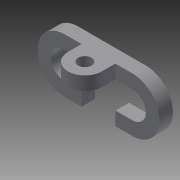
# Autodesk Inventor part: HW 2 Part 4
Saved by Autodesk Inventor 2015 SP1 (Build 190203100, 203)
## iProperties
Created: 2016-01-24
Part Number: HW 2 Part 4
Material: Generic
Document SubType Name: Modeling
Designer: melissa.roth
Density: 1 g/cm^3
Appearance: Default
Author: melissa.roth
Autodesk Inventor part; units mm, degrees
ref_plane "YZ Plane" through (0, 0, 0) normal (1, 0, 0) x (0, 1, 0)
ref_plane "XZ Plane" through (0, 0, 0) normal (0, 1, 0) x (-1, 0, 0)
ref_plane "XY Plane" through (0, 0, 0) normal (0, 0, 1) x (1, 0, 0)
sketch "Sketch1" plane through (0, 0, 0) normal (0, 0, 1) x (1, 0, 0)
  arc A0 (0, 12.7) -> (0, -12.7) centre (0, 0) ccw
  arc A1 (0, 25.4) -> (0, -25.4) centre (0, 0) ccw
  arc A2 (63.5, -12.7) -> (63.5, 12.7) centre (63.5, 0) ccw
  arc A3 (63.5, -25.4) -> (63.5, 25.4) centre (63.5, 0) ccw
  line L0 (0, 12.7) -> (63.5, 12.7)
  line L1 (0, -12.7) -> (63.5, -12.7)
  line L2 (0, 25.4) -> (63.5, 25.4)
  line L3 (0, -25.4) -> (63.5, -25.4)
  dimension "d0" = 25.4
  dimension "d1" = 50.8
  dimension "d2" = 25.4
  dimension "d3" = 50.8
  dimension "d4" = 63.5
  constraints: 8 end point, 8 point on circle, 4 centre point, 4 tangent, 3 coincident
  measures "d0" diameter of A0
  measures "d1" diameter of A1
  measures "d2" diameter of A2
  measures "d3" diameter of A3
  measures "d4" distance of A2.centre point (0, 0)
extrude "Extrusion1" add sketch "Sketch1" along normal blind 12.7
sketch "Sketch2" plane through (0, 0, 12.7) normal (0, 0, 1) x (1, 0, 0)
  line L0 (0, -25.4) -> (63.5, -25.4) projected
  line L1 (31.75, -25.4) -> (31.75, -12.7)
  line L2 (0, -12.7) -> (63.5, -12.7) projected
  line L3 (47.625, -12.7) -> (47.625, -25.4)
  line L4 (95.25, -31.75) -> (95.25, -25.4)
  line L5 (15.875, -12.7) -> (15.875, -25.4)
  line L6 (15.875, -12.7) -> (47.625, -12.7)
  line L7 (15.875, -25.4) -> (47.625, -25.4)
  point P0 (0, 0)
  dimension "d8" = 15.875
  dimension "d9" = 15.875
  constraints: 12 end point, 5 point on line, 3 perpendicular, 2 collinear, 2 midpoint
  measures "d8" distance between parallel lines of L1 L3
  measures "d9" distance between parallel lines of L1 L5
extrude "Extrusion2" cut sketch "Sketch2" against normal blind 12.7
sketch "Sketch4" plane through (0, 25.4, 0) normal (0, 1, 0) x (1, 0, 0)
  line L0 (63.5, 0) -> (0, 0) projected
  circle A0 centre (31.75, -25.4) radius 6.35
  arc A1 (15.875, -25.4) -> (47.625, -25.4) centre (31.75, -25.4) ccw
  line L1 (15.875, -25.4) -> (15.875, -12.7)
  line L2 (0, -12.7) -> (15.875, -12.7) projected
  line L3 (47.625, -25.4) -> (47.625, -12.7)
  line L4 (0, -12.7) -> (63.5, -12.7) projected
  line L5 (31.75, 0) -> (31.75, -12.7)
  dimension "d15" = 12.7
  dimension "d16" = 31.75
  dimension "d17" = 25.4
  dimension "d20" = 0
  constraints: 6 end point, 2 centre point, 2 midpoint, 2 point on circle, 2 point on line, 2 vertical, 1 coincident
  measures "d15" diameter of A0
  measures "d16" diameter of A1
  measures "d17" distance from line of L0 A0.centre
  measures "d20" horizontal distance of L5.end A0.centre
extrude "Extrusion3" add sketch "Sketch4" against normal blind 12.7
body "Solid1"
